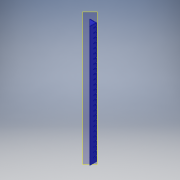
# Autodesk Inventor part: 3 x 3.25 steel with slits corner
Saved by Autodesk Inventor 2019 (Build 230136000, 136)
## iProperties
Created: 2017-12-19
Part Number: 3 x 3.25 steel with slits corner
Material: Steel
Document SubType Name: Modeling
Designer: torba
Density: 7.85 g/cm^3
Appearance: Blue - Wall Paint - Glossy
Author: torba
Autodesk Inventor part; units mm, degrees
ref_plane "YZ Plane" through (0, 0, 0) normal (1, 0, 0) x (0, 1, 0)
ref_plane "XZ Plane" through (0, 0, 0) normal (0, 1, 0) x (-1, 0, 0)
ref_plane "XY Plane" through (0, 0, 0) normal (0, 0, 1) x (1, 0, 0)
sketch "Sketch1" plane through (0, 0, 0) normal (0, 1, 0) x (-1, 0, 0)
  line L0 (0, 0) -> (0, -76.2)
  line L1 (0, -76.2) -> (76.2, -76.2)
  line L2 (76.2, -76.2) -> (76.2, -69.85)
  line L3 (76.2, -69.85) -> (6.35, -69.85)
  line L4 (6.35, -69.85) -> (6.35, 0)
  line L5 (6.35, 0) -> (0, 0)
  dimension "d0" = 76.2
  dimension "d1" = 76.2
  dimension "d2" = 6.35
  dimension "d3" = 6.35
  constraints: 12 end point, 5 perpendicular, 1 vertical
  measures "d0" distance of L0.start L0.end
  measures "d1" distance of L0.end L1.end
  measures "d2" distance between parallel lines of L1 L3
  measures "d3" distance between parallel lines of L0 L4
extrude "Extrusion1" add sketch "Sketch1" along normal blind 1358.9
fillet "Fillet1" radius 3.175 2 edges at (-6.35, 679.45, 0) (-76.2, 679.45, -69.85)
ref_plane "Work Plane2" through (-76.2, 0, -76.2) normal (-0.7071068, 0, -0.7071068) x (0, 1, 0)
sketch "Sketch4" plane through (-76.2, 0, -76.2) normal (-0.7071068, 0, -0.7071068) x (0, 1, 0)
  line L0 (0, 53.8815) -> (0, 0) projected
  line L1 (0, 0) -> (1358.9, 0) projected
  line L2 (1358.9, 53.8815) -> (1358.9, 0) projected
  line L3 (0, 53.8815) -> (1358.9, 53.8815) projected
  line L4 (0, 53.8815) -> (1358.9, 53.8815) projected
  line L5 (0, 53.8815) -> (50.8, 53.8815)
  line L6 (50.8, 53.8815) -> (58.7375, 53.8815)
  line L7 (58.7375, 53.8815) -> (58.7375, 28.4815)
  line L8 (58.7375, 28.4815) -> (50.8, 28.4815)
  line L9 (50.8, 28.4815) -> (50.8, 53.8815)
  dimension "d31" = 50.8
  dimension "d32" = 7.9375
  dimension "d33" = 25.4
  constraints: 10 end point, 2 parallel, 1 horizontal, 1 perpendicular, 1 point on line
  measures "d31" distance of L0.start L5.end
  measures "d32" distance of L7.end L8.end
  measures "d33" distance between parallel lines of L8 L3
extrude "Extrusion4" cut sketch "Sketch4" against normal blind 254 contours L3 L7 L8 L9
pattern_linear "Rectangular Pattern1" count 26 spacing 50.8 along (0, 1, 0) of "Extrusion4"
body "Solid1"
